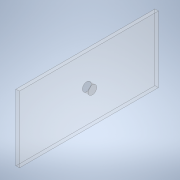
# Autodesk Inventor part: lid1
Saved by Autodesk Inventor 2021 (Build 250183000, 183)
## iProperties
Created: 2021-07-28
Part Number: lid1
Material: PMMA Plastic
Document SubType Name: Modeling
Designer: HP
Density: 1.188 g/cm^3
Appearance: Polycarbonate - Clear
Author: HP
Autodesk Inventor part; units mm, degrees
ref_plane "YZ Plane" through (0, 0, 0) normal (1, 0, 0) x (0, 1, 0)
ref_plane "XZ Plane" through (0, 0, 0) normal (0, 1, 0) x (-1, 0, 0)
ref_plane "XY Plane" through (0, 0, 0) normal (0, 0, 1) x (1, 0, 0)
sketch "Sketch1" plane through (0, 0, 0) normal (1, 0, 0) x (0, 1, 0)
  line L0 (6.35, 15.875) -> (-114.3, 15.875)
  line L1 (-114.3, 15.875) -> (-114.3, -236.5502)
  line L2 (-114.3, -236.5502) -> (6.35, -236.5502)
  line L3 (6.35, -236.5502) -> (6.35, 15.875)
  point P0 (0, 0)
  dimension "d0" = 120.65
  dimension "d1" = 252.4252
  constraints: 8 end point, 2 parallel, 1 horizontal, 1 perpendicular
  measures "d0" distance of L2.end L1.end
  measures "d1" distance of L1.end L0.end
extrude "Extrusion1" add sketch "Sketch1" along normal blind 6.35
sketch "Sketch2" plane through (6.35, 0, 0) normal (1, 0, 0) x (0, 0, -1)
  circle A0 centre (106.3625, -47.625) radius 7.9375
  point P0 (0, 0)
  constraints: 1 centre point
extrude "Extrusion2" add sketch "Sketch2" along normal blind 10.16
body "Solid1"
